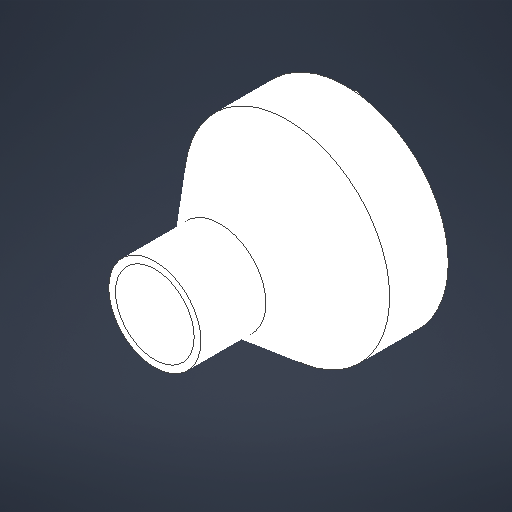
# Autodesk Inventor part: CAPSULA 1 MEDIDOR ESPORAS
Saved by Autodesk Inventor 2026.2 (Build 302298000, 298)
## iProperties
Created: 2025-12-31
Part Number: CAPSULA 1 MEDIDOR ESPORAS
Material: Genérico
Document SubType Name: Modeling
Designer: vicho
Density: 1 g/cm^3
Appearance: Valor por defecto
Author: vicho
Autodesk Inventor part; units mm, degrees
ref_plane "YZ Plane" through (0, 0, 0) normal (1, 0, 0) x (0, 1, 0)
ref_plane "XZ Plane" through (0, 0, 0) normal (0, 1, 0) x (-1, 0, 0)
sketch "Boceto1" plane through (0, 0, 0) normal (0, 0, 1) x (1, 0, 0)
  line L0 (0, 124.4663) -> (0, -121.5162) construction
  line L1 (-141.4483, 0) -> (147.5578, 0) construction
  circle A0 centre (0, 0) radius 17.5
  dimension "d0" = 35
  constraints: 4 end point, 2 horizontal, 2 point on line, 2 vertical, 1 centre point, 1 coincident
  measures "d0" diameter of A0
extrude "Extrusión1" add sketch "Boceto1" along normal blind 30
ref_plane "Plano de trabajo1" through (0, 0, -30) normal (0, 0, 1) x (1, 0, 0)
sketch "Boceto2" plane through (0, 0, -30) normal (0, 0, 1) x (1, 0, 0)
  circle A0 centre (0, 0) radius 42.5
  dimension "d4" = 85
  constraints: 1 centre point, 1 coincident
  measures "d4" diameter of A0
loft "Solevación1" add profiles "Boceto2" section 2 edges at (-17.5, 0, 0)
ref_plane "Plano de trabajo2" through (0, 0, -55) normal (0, 0, 1) x (1, 0, 0)
sketch "Boceto3" plane through (0, 0, -55) normal (0, 0, 1) x (1, 0, 0)
  circle A0 centre (0, 0) radius 42.5
  dimension "d10" = 85
  constraints: 1 centre point, 1 coincident
  measures "d10" diameter of A0
loft "Solevación2" add profiles "Boceto3" section 2 edges at (-42.5, 0, -30)
shell "Vaciado1" thickness 3 outward yes removed faces 2 at (-10.6049, 7.3037, -55) at (4.3663, -1.0762, 30)
sketch "Boceto4" plane through (0, 0, -55) normal (0, 0, -1) x (-1, 0, 0)
  circle A0 centre (0, 0) radius 44.5
  circle A1 centre (0, 0) radius 42.5
  line L0 (-2.5, 42.4264) -> (-2.5, 36.4244)
  line L1 (-2.5, 36.4244) -> (2.5, 36.4244)
  line L2 (2.5, 36.4244) -> (2.5, 42.4264)
  line L3 (-61.729, 0) -> (90.2911, 0) construction
  line L4 (0, 48.1461) -> (0, -48.1461) construction
  circle A2 centre (0, 0) radius 37 construction
  circle A3 centre (0, 0) radius 40 construction
  circle A4 centre (0, 0) radius 38.5 construction
  arc A5 (-2.5, 38.5) -> (2.5, 38.5) centre (0, 38.5) ccw
  line L5 (-35.4923, -23.3783) -> (-30.2945, -20.3773)
  arc A6 (-32.092, -21.4151) -> (-34.592, -17.0849) centre (-33.342, -19.25) ccw
  line L6 (-32.7945, -16.0472) -> (-37.9923, -19.0481)
  line L7 (37.9923, -19.0481) -> (32.7945, -16.0472)
  arc A7 (34.592, -17.0849) -> (32.092, -21.4151) centre (33.342, -19.25) ccw
  line L8 (30.2945, -20.3773) -> (35.4923, -23.3783)
  dimension "d21" = 77
  dimension "d16" = 85
  dimension "d17" = 74
  dimension "d18" = 80
  dimension "d19" = 5
  dimension "d20" = 6.002
  dimension "d22" = 5
  dimension "d25" = 360
  constraints: 18 end point, 9 point on line, 8 point on circle, 7 centre point, 6 coincident, 2 midpoint, 2 vertical, 1 horizontal, 1 perpendicular, 1 tangent, 1 vertical alignment, 34 other
  measures "d16" diameter of A1
  measures "d17" diameter of A2
  measures "d18" diameter of A3
  measures "d19" distance of L1.end L0.end
  measures "d20" distance of L0.start L0.end
  measures "d22" distance between parallel lines of L2 L0
extrude "Extrusión2" add sketch "Boceto4" against normal blind 3 contours L2 A5 L1 L0 A1 | A1 L8 A7 L7 | L6 A6 L5 A1 | A5 L1
ref_plane "Plano de trabajo3" through (0, 0, -60) normal (0, 0, 1) x (1, 0, 0)
sketch "Boceto5" plane through (0, 0, -60) normal (0, 0, 1) x (1, 0, 0)
  line L0 (0, 47.3974) -> (0, -47.5019) construction
  line L1 (54.9107, 0) -> (-68.9978, 0) construction
  circle A0 centre (0, 0) radius 38.5 construction
  circle A1 centre (0, 38.5) radius 2.5
  circle A2 centre (-33.342, -19.25) radius 2.5
  circle A3 centre (33.342, -19.25) radius 2.5
  dimension "d30" = 77
  dimension "d31" = 5
  dimension "d34" = 360
  constraints: 4 end point, 3 centre point, 3 point on line, 2 coincident, 1 horizontal, 1 vertical, 1 vertical alignment, 9 other
  measures "d31" diameter of A1
extrude "Extrusión3" add sketch "Boceto5" along normal blind 5
sketch "Boceto6" plane through (33.342, -19.25, -60) normal (0, 0, -1) x (-1, 0, 0)
  circle A0 centre (0, 0) radius 1.525
  circle A1 centre (0, 0) radius 2.5 construction
  circle A2 centre (66.684, 0) radius 1.525
  circle A3 centre (33.342, 57.75) radius 1.525
  point P0 (33.342, 19.25)
  dimension "d38" = 3.05
  dimension "d39" = 0.975
  dimension "d42" = 360
  constraints: 3 centre point, 7 other
  measures "d38" diameter of A0
  measures "d39" radial gap between concentric circles of A1 A0
extrude "Extrusión4" cut sketch "Boceto6" against normal blind 5
